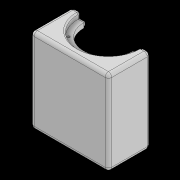
# Autodesk Inventor part: tonguev2
Saved by Autodesk Inventor 2022 (Build 260153000, 153)
## iProperties
Created: 2022-06-28
Part Number: tonguev2
Material: Generic
Document SubType Name: Modeling
Designer: Fuzzyfish
Density: 1 g/cm^3
Appearance: Default
Author: Fuzzyfish
Autodesk Inventor part; units mm, degrees
ref_plane "YZ Plane" through (0, 0, 0) normal (1, 0, 0) x (0, 1, 0)
ref_plane "XZ Plane" through (0, 0, 0) normal (0, 1, 0) x (-1, 0, 0)
sketch "Sketch1" plane through (0, 0, 0) normal (0, 1, 0) x (-1, 0, 0)
  line L0 (0, 0) -> (105, 0)
  line L1 (105, 0) -> (105, -105)
  line L2 (105, -105) -> (0, -105)
  line L3 (0, -105) -> (0, 0)
  circle A0 centre (52.5, -52.5) radius 36.5
  dimension "d0" = 105
  dimension "d1" = 105
  dimension "d2" = 52.5
  dimension "d3" = 52.5
  dimension "d4" = 73
  constraints: 8 end point, 2 parallel, 1 centre point, 1 horizontal, 1 perpendicular
  measures "d0" distance of L0.end L1.end
  measures "d1" distance of L1.end L2.end
  measures "d2" distance from line of L1 A0.centre
  measures "d3" distance from line of L0 A0.centre
  measures "d4" diameter of A0
extrude "Extrusion1" add sketch "Sketch1" along normal blind 7
sketch "Sketch3" plane through (-105, 0, 0) normal (0, 0, 1) x (1, 0, 0)
  line L0 (105, 7) -> (0, 7) projected
  line L1 (0, 7) -> (105, 7)
  line L2 (105, 7) -> (105, -105)
  line L3 (105, -105) -> (0, -105)
  line L4 (0, -105) -> (0, 7)
  line L5 (0, 0) -> (105, 0) projected
  dimension "d7" = 105
  constraints: 8 end point, 2 parallel, 1 horizontal, 1 perpendicular
  measures "d7" distance between parallel lines of L5 L3
extrude "Extrusion2" add sketch "Sketch3" along normal blind 5
sketch "Sketch4" plane through (-105, 0, -105) normal (-1, 0, 0) x (0, 0, 1)
  line L0 (0, 0) -> (0, 7) projected
  line L1 (0, 7) -> (110, 7)
  line L2 (110, 7) -> (110, -105)
  line L3 (110, -105) -> (0, -105)
  line L4 (0, -105) -> (0, 7)
  point P0 (105, 0)
  constraints: 8 end point, 2 parallel, 1 horizontal, 1 perpendicular
extrude "Extrusion3" add sketch "Sketch4" along normal blind 5
sketch "Sketch6" plane through (0, 0, -105) normal (0, 0, -1) x (-1, 0, 0)
  line L0 (0, 7) -> (110, 7) projected
  line L1 (110, -105) -> (110, 7) projected
  line L2 (0, 7) -> (110, 7)
  line L3 (110, 7) -> (110, -105)
  line L4 (110, -105) -> (0, -105)
  line L5 (0, -105) -> (0, 7)
  point P0 (0, 0)
  constraints: 8 end point, 2 parallel, 1 horizontal, 1 perpendicular
extrude "Extrusion4" add sketch "Sketch6" along normal blind 5
sketch "Sketch7" plane through (0, -105, 0) normal (1, 0, 0) x (0, 0, -1)
  line L0 (-5, 0) -> (-5, 112) projected
  line L1 (105, 0) -> (110, 0) projected
  line L2 (-5, 112) -> (110, 112)
  line L3 (110, 112) -> (110, 0)
  line L4 (110, 0) -> (-5, 0)
  line L5 (-5, 0) -> (-5, 112)
  point P0 (0, 105)
  constraints: 8 end point, 2 parallel, 1 horizontal, 1 perpendicular
extrude "Extrusion5" add sketch "Sketch7" along normal blind 5
sketch "Sketch8" plane through (-110, -105, -110) normal (0, -1, 0) x (1, 0, 0)
  line L0 (0, 115) -> (115, 115) projected
  line L1 (0, 0) -> (115, 0) projected
  line L2 (0, 115) -> (115, 115)
  line L3 (115, 115) -> (115, 0)
  line L4 (115, 0) -> (0, 0)
  line L5 (0, 0) -> (0, 115)
  point P0 (110, 110)
  constraints: 8 end point, 2 parallel, 1 horizontal, 1 perpendicular
extrude "Extrusion6" add sketch "Sketch8" along normal blind 5
sketch "Sketch9" plane through (0, 7, 0) normal (0, 1, 0) x (1, 0, 0)
  line L0 (-110, -5) -> (-110, 110) projected
  line L1 (-110, -5) -> (5, -5) projected
  line L2 (5, 110) -> (5, -5) projected
  line L3 (-110, 110) -> (5, 110) projected
  circle A0 centre (-52.5, 52.5) radius 36.5 projected
  line L4 (-110, -5) -> (-110, 110) projected
  line L5 (-110, 110) -> (5, 110) projected
  line L6 (-110, -5) -> (5, -5)
  line L7 (5, -5) -> (5, 110)
  line L8 (5, 110) -> (-110, 110)
  line L9 (-110, 110) -> (-110, -5)
  circle A1 centre (-52.5, 52.5) radius 45
  dimension "d18" = 90
  constraints: 8 end point, 2 parallel, 1 centre point, 1 coincident, 1 horizontal, 1 perpendicular
  measures "d18" diameter of A1
extrude "Extrusion7" add sketch "Sketch9" along normal blind 8 contours L0 L3 L2 L1
sketch "Sketch10" plane through (-52.5, 7, -52.5) normal (0, 1, 0) x (1, 0, 0)
  line L0 (57.5, -57.5) -> (-57.5, -57.5) construction
  line L1 (57.5, 57.5) -> (57.5, -57.5) construction
  line L2 (-57.5, -57.5) -> (57.5, 57.5) construction
  line L3 (57.5, 57.5) -> (-57.5, 57.5) construction
  line L4 (-57.5, 57.5) -> (57.5, -57.5) construction
  circle A0 centre (0, 0) radius 41.75 construction
  circle A1 centre (-29.5217, -29.5217) radius 1.9
  circle A2 centre (-29.5217, 29.5217) radius 1.9
  circle A3 centre (29.5217, 29.5217) radius 1.9
  circle A4 centre (29.5217, -29.5217) radius 1.9
  line L5 (0, -57.5) -> (0, 57.5) construction
  point P0 (52.5, -52.5)
  dimension "d21" = 3.8
  dimension "d22" = 83.5
  dimension "d23" = 3.8
  dimension "d24" = 3.8
  dimension "d25" = 3.8
  dimension "d26" = 45
  constraints: 8 end point, 5 centre point, 4 point on circle, 4 point on line, 3 midpoint, 2 perpendicular
  measures "d21" diameter of A1
  measures "d22" diameter of A0
  measures "d23" diameter of A2
  measures "d24" diameter of A3
  measures "d25" diameter of A4
  measures "d26" angle of L5 L2
extrude "Extrusion8" cut sketch "Sketch10" against normal blind 5
ref_plane "Work Plane1" through (0, 0, -52.5) normal (0, 0, -1) x (-1, 0, 0)
fillet "Fillet2" radius 5 12 edges at (-105, -105, -52.5) (-105, -52.5, -105) (-52.5, -105, -105) (0, -52.5, -105) (0, -52.5, 0) (-52.5, -105, 0) (0, -105, -52.5) (-105, -52.5, 0) (-52.5, 0, -105) (0, 0, -52.5) (-52.5, 0, 0) (-105, 0, -52.5)
fillet "Fillet3" radius 5 12 edges at (-52.5, 15, 5) (-110, 15, -52.5) (-110, -47.5, 5) (-110, -110, -52.5) (-110, -47.5, -110) (-52.5, 15, -110) (5, 15, -52.5) (5, -47.5, 5) (5, -47.5, -110) (-52.5, -110, -110) (5, -110, -52.5) (-52.5, -110, 5)
split "Split2" plane through (0, 0, -52.5) removes the side toward (0, 0, -1)
chamfer "Chamfer1" distance 2 angle 45 1 edges at (-52.5, 15, -7.5)
sketch "Sketch15" plane through (0, 0, -52.5) normal (0, 0, -1) x (-1, 0, 0)
  arc A0 (-5, -105) -> (0, -110) centre (0, -105) ccw projected
  line L0 (-5, -105) -> (-5, 10) projected
  arc A1 (0, 15) -> (-5, 10) centre (0, 10) ccw projected
  arc A2 (5, 0) -> (0, -5) centre (5, -5) ccw projected
  line L1 (0, -5) -> (0, -100) projected
  arc A3 (0, -100) -> (5, -105) centre (5, -100) ccw projected
  line L2 (5, -105) -> (100, -105) projected
  arc A4 (100, -105) -> (105, -100) centre (100, -100) ccw projected
  line L3 (105, -100) -> (105, -5) projected
  arc A5 (105, -5) -> (100, 0) centre (100, -5) ccw projected
  arc A6 (110, 10) -> (105, 15) centre (105, 10) ccw projected
  line L4 (110, 10) -> (110, -105) projected
  arc A7 (105, -110) -> (110, -105) centre (105, -105) ccw projected
  line L5 (105, -110) -> (0, -110) projected
  line L6 (100, 0) -> (89, 0) projected
  line L7 (89, 0) -> (89, 7) projected
  line L8 (89, 7) -> (97.5, 7) projected
  line L9 (97.5, 7) -> (97.5, 13) projected
  line L10 (97.5, 13) -> (99.5, 15) projected
  line L11 (99.5, 15) -> (105, 15) projected
  line L12 (0, 15) -> (5.5, 15) projected
  line L13 (5.5, 15) -> (7.5, 13) projected
  line L14 (7.5, 13) -> (7.5, 7) projected
  line L15 (7.5, 7) -> (16, 7) projected
  line L16 (16, 7) -> (16, 0) projected
  line L17 (16, 0) -> (5, 0) projected
  line L18 (4.9615, 13.7) -> (0, 13.7)
  arc A8 (0, 13.7) -> (-3.7, 10) centre (0, 10) ccw
  line L19 (-3.7, 10) -> (-3.7, -105)
  arc A9 (-3.7, -105) -> (0, -108.7) centre (0, -105) ccw
  line L20 (0, -108.7) -> (105, -108.7)
  arc A10 (105, -108.7) -> (108.7, -105) centre (105, -105) ccw
  line L21 (108.7, -105) -> (108.7, 10)
  arc A11 (108.7, 10) -> (105, 13.7) centre (105, 10) ccw
  line L22 (105, 13.7) -> (100.0385, 13.7)
  line L23 (100.0385, 13.7) -> (98.8, 12.4615)
  line L24 (98.8, 12.4615) -> (98.8, 5.7)
  line L25 (98.8, 5.7) -> (90.3, 5.7)
  line L26 (90.3, 5.7) -> (90.3, 1.3)
  line L27 (90.3, 1.3) -> (100, 1.3)
  arc A12 (106.3, -5) -> (100, 1.3) centre (100, -5) ccw
  line L28 (106.3, -5) -> (106.3, -100)
  arc A13 (100, -106.3) -> (106.3, -100) centre (100, -100) ccw
  line L29 (100, -106.3) -> (5, -106.3)
  arc A14 (-1.3, -100) -> (5, -106.3) centre (5, -100) ccw
  line L30 (-1.3, -100) -> (-1.3, -5)
  arc A15 (5, 1.3) -> (-1.3, -5) centre (5, -5) ccw
  line L31 (5, 1.3) -> (14.7, 1.3)
  line L32 (14.7, 1.3) -> (14.7, 5.7)
  line L33 (14.7, 5.7) -> (6.2, 5.7)
  line L34 (6.2, 5.7) -> (6.2, 12.4615)
  line L35 (6.2, 12.4615) -> (4.9615, 13.7)
  dimension "d52" = 1.3
  constraints: 36 end point, 16 point on circle, 8 centre point, 25 other
  measures "d52" distance between parallel lines of L12 L18
extrude "Extrusion11" add sketch "Sketch15" along normal blind 3 contours L35 L34 L33 L32 L31 A15 L30 A14 L29 A13 L28 A12 L27 L26 L25 L24 L23 L22 A11 L21 A10 L20 A9 L19 A8 L18
sketch "Sketch16" plane through (-110, -110, -110) normal (0, -1, 0) x (1, 0, 0)
  line L0 (5, 57.5) -> (110, 57.5) projected
  line L1 (5, 57.5) -> (5, 54.5) projected
  line L2 (110, 54.5) -> (5, 54.5) projected
  line L3 (110, 57.5) -> (110, 54.5) projected
  line L4 (110, 54.5) -> (5, 54.5) projected
  circle A0 centre (57.5, 56) radius 2
  line L5 (5, 57.5) -> (110, 57.5) projected
  point P0 (110, 110)
  point P1 (58.8229, 54.5)
  point P2 (56.1771, 54.5)
  dimension "d54" = 4
  dimension "d55" = 105
  dimension "d56" = 52.5
  dimension "d59" = 1.5
  constraints: 1 centre point
  measures "d54" diameter of A0
  measures "d55" distance of L0.start L0.end
  measures "d56" distance from line of L3 A0.centre
  measures "d59" distance from line of L0 A0.centre
extrude "Extrusion13" cut sketch "Sketch16" against normal blind 10 contours A0 L0 | L0 A0 L2
equation "\"d2\" = 0.5 * d1"
equation "\"d3\" = 0.5 * d0"
equation "\"d23\" = d21"
equation "\"d24\" = d23"
equation "\"d25\" = d24"
equation "\"d56\" = 0.5 * d55"
body "Solid1"
